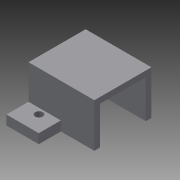
# Autodesk Inventor part: gear_bracket
Saved by Autodesk Inventor 2015 (Build 190159000, 159)
## iProperties
Created: 2014-10-24
Part Number: gear_bracket
Material: Generic
Document SubType Name: Modeling
Designer: Colin
Density: 1 g/cm^3
Appearance: Default
Author: Colin
Autodesk Inventor part; units mm, degrees
ref_plane "YZ Plane" through (0, 0, 0) normal (1, 0, 0) x (0, 1, 0)
ref_plane "XZ Plane" through (0, 0, 0) normal (0, 1, 0) x (-1, 0, 0)
ref_plane "XY Plane" through (0, 0, 0) normal (0, 0, 1) x (1, 0, 0)
sketch "Sketch3" plane through (0, 0, 0) normal (1, 0, 0) x (0, 1, 0)
  line L0 (0, 0) -> (0, -7.3)
  line L1 (0, 0) -> (2.5, 0)
  line L2 (2.5, 0) -> (2.5, -5.8)
  line L3 (2.5, -5.8) -> (11.5, -5.8)
  line L4 (0, -13.3) -> (11.5, -13.3) construction
  line L5 (0, -26.6) -> (2.5, -26.6)
  line L6 (2.5, -26.6) -> (2.5, -20.8)
  line L7 (2.5, -20.8) -> (11.5, -20.8)
  line L8 (11.5, -5.8) -> (11.5, -20.8)
  line L9 (0, -7.3) -> (10, -7.3)
  line L10 (10, -7.3) -> (10, -19.3)
  line L11 (10, -19.3) -> (0, -19.3)
  line L12 (0, -19.3) -> (0, -26.6)
  dimension "d10" = 26.6
  dimension "d12" = 2.5
  dimension "d13" = 5.8
  dimension "d14" = 11.5
  dimension "d15" = 1.5
  dimension "d16" = 1.5
  dimension "d17" = 1.5
  constraints: 26 end point, 4 horizontal, 4 vertical, 3 symmetric about line, 1 parallel, 1 perpendicular
  measures "d10" distance of L0.start L5.start
  measures "d12" distance of L0.start L1.end
  measures "d13" distance of L1.end L2.end
  measures "d14" distance from line of L3.end L0
  measures "d15" distance between parallel lines of L3 L9
  measures "d16" distance between parallel lines of L8 L10
  measures "d17" distance between parallel lines of L7 L11
extrude "Extrusion1" add sketch "Sketch3" along normal blind 17.3
sketch "Sketch5" plane through (0, 0, -26.6) normal (0, -1, 0) x (1, 0, 0)
  line L0 (0, 0) -> (8.5, 0) construction
  line L1 (8.5, 0) -> (8.5, 5.8) construction
  line L2 (8.5, 5.8) -> (0, 5.8) construction
  line L3 (0, 5.8) -> (0, 0) construction
  line L4 (8.5, 0) -> (17.3, 0)
  line L5 (17.3, 0) -> (17.3, 5.8)
  line L6 (17.3, 5.8) -> (8.5, 5.8)
  line L7 (8.5, 5.8) -> (8.5, 0)
  line L8 (0, 19.3) -> (0, 7.3) projected
  line L9 (0, 13.3) -> (17.3, 13.3) construction
  line L10 (8.5, 26.6) -> (8.5, 20.8) construction
  line L11 (8.5, 26.6) -> (17.3, 26.6)
  line L12 (17.3, 26.6) -> (17.3, 20.8)
  line L13 (17.3, 20.8) -> (8.5, 20.8)
  line L14 (8.5, 20.8) -> (8.5, 26.6)
  point P0 (0, 26.6)
  dimension "d22" = 5.8
  dimension "d23" = 8.5
  constraints: 28 end point, 5 symmetric about line, 4 parallel, 3 horizontal, 2 perpendicular, 1 midpoint
  measures "d22" distance of L2.end L0.start
  measures "d23" distance of L1.end L2.end
extrude "Extrusion2" cut sketch "Sketch5" against normal through all
sketch "Sketch6" plane through (0, 0, -7.3) normal (0, -1, 0) x (1, 0, 0)
  circle A0 centre (4.25, 3) radius 1.016
  line L0 (0, 7.3) -> (0, 0) projected
  line L1 (0, 0) -> (0, -12) projected
  line L2 (0, -6) -> (17.3, -6) construction
  line L3 (17.3, -13.5) -> (17.3, 1.5) projected
  circle A1 centre (4.25, -15) radius 1.016
  dimension "d26" = 2.032
  dimension "d27" = 4.25
  dimension "d28" = 18
  constraints: 2 centre point, 2 end point, 2 midpoint, 1 symmetric about line, 1 other
  measures "d26" diameter of A0
  measures "d27" distance from line of L0 A0.centre
  measures "d28" distance of A1.centre A0.centre
extrude "Extrusion3" cut sketch "Sketch6" against normal through all
body "Solid1"
